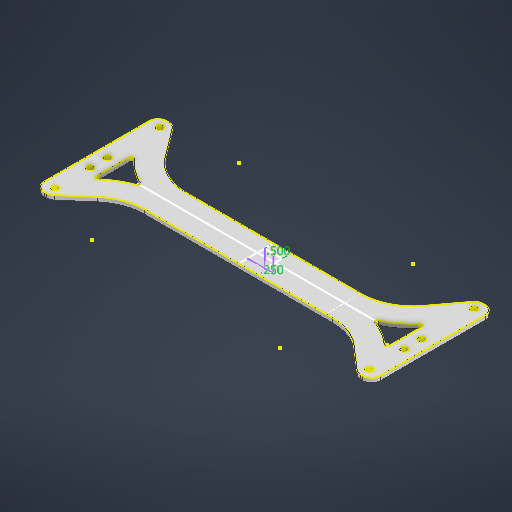
# Autodesk Inventor part: Lady Brown Arm Brace
Saved by Autodesk Inventor 2025 (Build 290162000, 162)
## iProperties
Created: 2024-12-31
Part Number: Lady Brown Arm Brace
Material: Generic
Document SubType Name: Modeling
Designer: Juan
Density: 1 g/cm^3
Appearance: Default
Author: Juan
Autodesk Inventor part; units mm, degrees
ref_plane "YZ Plane" through (0, 0, 0) normal (1, 0, 0) x (0, 1, 0)
ref_plane "XZ Plane" through (0, 0, 0) normal (0, 1, 0) x (-1, 0, 0)
ref_plane "XY Plane" through (0, 0, 0) normal (0, 0, 1) x (1, 0, 0)
sketch "Sketch1" plane through (0, 0, 0) normal (0, 1, 0) x (-1, 0, 0)
  line L0 (0, 0) -> (-114.3, 0)
  line L1 (0, 0) -> (114.3, 0)
  circle A0 centre (-114.3, 0) radius 2.3241
  circle A1 centre (114.3, 0) radius 2.3241
  line L2 (-114.3, 0) -> (-114.3, 12.7)
  line L3 (114.3, 0) -> (114.3, 12.7)
  circle A2 centre (114.3, 12.7) radius 2.3241
  circle A3 centre (-114.3, 12.7) radius 2.3241
  line L4 (114.3, 0) -> (122.2375, 0)
  line L5 (-114.3, 0) -> (-122.2375, 0)
  line L6 (-114.3, 12.7) -> (-122.2375, 12.7)
  line L7 (114.3, 12.7) -> (122.2375, 12.7)
  line L8 (-114.3, 0) -> (-114.3, -6.35)
  line L9 (-114.3, 12.7) -> (-114.3, 19.05)
  line L10 (114.3, 0) -> (114.3, -6.35)
  line L11 (114.3, 12.7) -> (114.3, 19.05)
  line L12 (122.2375, -6.35) -> (-122.2375, -6.35)
  line L13 (-122.2375, -6.35) -> (-122.2375, 19.05)
  line L14 (-122.2375, 19.05) -> (122.2375, 19.05)
  line L15 (122.2375, 19.05) -> (122.2375, -6.35)
  dimension "d0" = 114.3
  dimension "d1" = 114.3
  dimension "d2" = 4.6482
  dimension "d3" = 4.6482
  dimension "d4" = 12.7
  dimension "d5" = 12.7
  dimension "d6" = 4.6482
  dimension "d7" = 4.6482
  dimension "d8" = 7.9375
  dimension "d9" = 7.9375
  dimension "d10" = 6.35
  dimension "d11" = 6.35
  constraints: 32 end point, 7 horizontal, 6 vertical, 4 centre point, 4 coincident, 2 parallel, 1 perpendicular
  measures "d0" distance of L0.start L0.end
  measures "d1" distance of L0.start L1.end
  measures "d2" diameter of A0
  measures "d3" diameter of A1
  measures "d4" distance of L2.start L2.end
  measures "d5" distance of L3.start L3.end
  measures "d6" diameter of A2
  measures "d7" diameter of A3
  measures "d8" distance of L3.start L4.end
  measures "d9" distance of L2.start L5.end
  measures "d10" distance of L2.start L8.end
  measures "d11" distance of L6.start L9.end
extrude "Extrusion1" add sketch "Sketch1" along normal blind 3.175 contours L1 A1 L10 L12 L8 A0 L0 | L0 A0 L2 A3 L9 L14 L11 A2 L3 A1 L1 | A0 L5 L13 L6 A3 L2 | L8 L12 L13 L5 A0 | L3 A2 L7 L15 L4 A1 | A1 L4 L15 L12 L10 | L6 L13 L14 L9 A3 | L11 L14 L15 L7 A2
sketch "Sketch2" plane through (0, 3.175, 0) normal (0, 1, 0) x (1, 0, 0)
  circle A0 centre (114.3, -12.7) radius 2.3241 projected
  line L0 (0, 0) -> (0, -19.05)
  line L1 (-122.2375, -19.05) -> (122.2375, -19.05) projected
  line L2 (114.3, -12.7) -> (114.3, -38.1)
  circle A1 centre (114.3, -38.1) radius 2.3241
  line L3 (122.2375, -19.05) -> (107.95, -19.05)
  line L4 (107.95, -19.05) -> (107.95, -44.45)
  line L5 (107.95, -44.45) -> (122.2375, -44.45)
  line L6 (122.2375, -44.45) -> (122.2375, -19.05)
  circle A2 centre (114.3, 0) radius 2.3241 projected
  line L7 (114.3, 0) -> (114.3, 38.1)
  circle A3 centre (114.3, 38.1) radius 2.3241
  line L8 (122.2375, 6.35) -> (-122.2375, 6.35) projected
  line L9 (122.2375, 6.35) -> (107.95, 6.35)
  line L10 (107.95, 6.35) -> (107.95, 44.45)
  line L11 (107.95, 44.45) -> (122.2375, 44.45)
  line L12 (122.2375, 44.45) -> (122.2375, 6.35)
  line L13 (122.2375, -19.05) -> (122.2375, 6.35) projected
  circle A4 centre (-114.3, -38.1) radius 2.3241
  line L14 (-107.95, -19.05) -> (-107.95, -44.45)
  line L15 (-107.95, -44.45) -> (-122.2375, -44.45)
  line L16 (-122.2375, -44.45) -> (-122.2375, -19.05)
  circle A5 centre (-114.3, 38.1) radius 2.3241
  line L17 (-107.95, 6.35) -> (-107.95, 44.45)
  line L18 (-107.95, 44.45) -> (-122.2375, 44.45)
  line L19 (-122.2375, 44.45) -> (-122.2375, 6.35)
  line L20 (-122.2375, 6.35) -> (-122.2375, -19.05) projected
  dimension "d14" = 25.4
  dimension "d15" = 14.2875
  dimension "d16" = 25.4
  dimension "d17" = 38.1
  dimension "d18" = 4.6482
  dimension "d19" = 14.2875
  dimension "d20" = 38.1
  constraints: 34 end point, 8 symmetric about line, 4 centre point, 4 parallel, 2 coincident, 2 horizontal, 2 perpendicular, 2 vertical, 1 midpoint, 2 other
  measures "d14" distance of L2.start L2.end
  measures "d15" distance of L5.end L4.end
  measures "d16" distance of L5.end L1.end
  measures "d17" distance of L7.start L7.end
  measures "d18" diameter of A3
  measures "d19" distance of L10.end L11.end
  measures "d20" distance of L11.end L8.start
extrude "Extrusion2" add sketch "Sketch2" against normal blind 3.175 contours L1 L14 L15 L16 | L19 L18 L17 L8 | L1 L6 L5 L4 | L10 L11 L12 L8
fillet "Fillet1" radius 6.35 8 edges at (122.2375, 1.5875, 44.45) (107.95, 1.5875, 44.45) (122.2375, 1.5875, -44.45) (107.95, 1.5875, -44.45) (-107.95, 1.5875, 44.45) (-122.2375, 1.5875, 44.45) (-122.2375, 1.5875, -44.45) (-107.95, 1.5875, -44.45)
sketch "Sketch3" plane through (0, 3.175, 0) normal (0, 1, 0) x (1, 0, 0)
  line L0 (-107.95, -19.05) -> (107.95, -19.05) projected
  line L1 (107.95, -19.05) -> (107.95, -38.1) projected
  line L2 (-107.95, -38.1) -> (-107.95, -19.05) projected
  arc A0 (-114.3, -44.45) -> (-107.95, -38.1) centre (-114.3, -38.1) ccw projected
  arc A1 (107.95, -38.1) -> (114.3, -44.45) centre (114.3, -38.1) ccw projected
  line L3 (-107.95, -19.05) -> (107.95, -19.05) projected
  line L4 (107.95, -19.05) -> (82.55, -19.05)
  line L5 (82.55, -19.05) -> (110.1475, -42.9041)
  line L6 (0, 0) -> (0, -19.05)
  line L7 (107.95, 6.35) -> (-107.95, 6.35) projected
  line L8 (107.95, 6.35) -> (82.55, 6.35)
  arc A2 (114.3, 44.45) -> (107.95, 38.1) centre (114.3, 38.1) ccw projected
  line L9 (107.95, 38.1) -> (107.95, 6.35) projected
  line L10 (-107.95, 6.35) -> (-107.95, 38.1) projected
  arc A3 (-107.95, 38.1) -> (-114.3, 44.45) centre (-114.3, 38.1) ccw projected
  line L11 (82.55, 6.35) -> (109.22, 41.91)
  line L12 (-82.55, -19.05) -> (-110.1475, -42.9041)
  line L13 (-82.55, 6.35) -> (-109.22, 41.91)
  dimension "d24" = 25.4
  constraints: 14 end point, 4 symmetric about line, 2 point on circle, 2 point on line, 2 tangent, 1 midpoint
  measures "d24" distance of L0.end L4.end
extrude "Extrusion3" add sketch "Sketch3" against normal blind 3.175
fillet "Fillet2" radius 38.1 2 edges at (82.55, 1.5875, -6.35) (-82.55, 1.5875, -6.35)
fillet "Fillet3" radius 38.1 2 edges at (-82.55, 1.5875, 19.05) (82.55, 1.5875, 19.05)
sketch "Sketch4" plane through (0, 3.175, 0) normal (0, 1, 0) x (1, 0, 0)
  circle A0 centre (-114.3, 38.1) radius 2.3241 projected
  circle A1 centre (114.3, -38.1) radius 2.3241 projected
  circle A2 centre (-114.3, -38.1) radius 2.3241 projected
  circle A3 centre (114.3, 38.1) radius 2.3241 projected
  arc A4 (-109.22, 41.91) -> (-114.3, 44.45) centre (-114.3, 38.1) ccw projected
  line L0 (-114.3, 44.45) -> (-115.8875, 44.45) projected
  arc A5 (-115.8875, 44.45) -> (-122.2375, 38.1) centre (-115.8875, 38.1) ccw projected
  line L1 (-122.2375, 38.1) -> (-122.2375, -38.1) projected
  arc A6 (-122.2375, -38.1) -> (-115.8875, -44.45) centre (-115.8875, -38.1) ccw projected
  line L2 (-115.8875, -44.45) -> (-114.3, -44.45) projected
  arc A7 (-114.3, -44.45) -> (-110.1475, -42.9041) centre (-114.3, -38.1) ccw projected
  line L3 (-110.1475, -42.9041) -> (-93.2809, -28.3253) projected
  arc A8 (-68.3661, -19.05) -> (-93.2809, -28.3253) centre (-68.3661, -57.15) ccw projected
  line L4 (-68.3661, -19.05) -> (68.3661, -19.05) projected
  arc A9 (93.2809, -28.3253) -> (68.3661, -19.05) centre (68.3661, -57.15) ccw projected
  line L5 (93.2809, -28.3253) -> (110.1475, -42.9041) projected
  arc A10 (110.1475, -42.9041) -> (114.3, -44.45) centre (114.3, -38.1) ccw projected
  line L6 (114.3, -44.45) -> (115.8875, -44.45) projected
  arc A11 (115.8875, -44.45) -> (122.2375, -38.1) centre (115.8875, -38.1) ccw projected
  line L7 (122.2375, -38.1) -> (122.2375, 38.1) projected
  arc A12 (122.2375, 38.1) -> (115.8875, 44.45) centre (115.8875, 38.1) ccw projected
  line L8 (115.8875, 44.45) -> (114.3, 44.45) projected
  arc A13 (114.3, 44.45) -> (109.22, 41.91) centre (114.3, 38.1) ccw projected
  line L9 (109.22, 41.91) -> (93.98, 21.59) projected
  arc A14 (63.5, 6.35) -> (93.98, 21.59) centre (63.5, 44.45) ccw projected
  line L10 (63.5, 6.35) -> (-63.5, 6.35) projected
  arc A15 (-93.98, 21.59) -> (-63.5, 6.35) centre (-63.5, 44.45) ccw projected
  line L11 (-93.98, 21.59) -> (-109.22, 41.91) projected
  circle A16 centre (114.3, 0) radius 2.3241 projected
  circle A17 centre (-114.3, 0) radius 2.3241 projected
  circle A18 centre (-114.3, -12.7) radius 2.3241 projected
  circle A19 centre (114.3, -12.7) radius 2.3241 projected
  line L12 (-63.5, -9.174) -> (63.5, -9.174)
  arc A20 (63.5, -9.174) -> (106.3992, 12.2756) centre (63.5, 44.45) ccw
  line L13 (106.3992, 12.2756) -> (106.7135, 12.6946)
  line L14 (106.7135, 12.6946) -> (106.7135, -19.4165)
  line L15 (106.7135, -19.4165) -> (103.4325, -16.5806)
  arc A21 (103.4325, -16.5806) -> (68.3661, -3.526) centre (68.3661, -57.15) ccw
  line L16 (68.3661, -3.526) -> (-68.3661, -3.526)
  arc A22 (-68.3661, -3.526) -> (-103.4325, -16.5806) centre (-68.3661, -57.15) ccw
  line L17 (-103.4325, -16.5806) -> (-106.7135, -19.4165)
  line L18 (-106.7135, -19.4165) -> (-106.7135, 12.6946)
  line L19 (-106.7135, 12.6946) -> (-106.3992, 12.2756)
  arc A23 (-106.3992, 12.2756) -> (-63.5, -9.174) centre (-63.5, 44.45) ccw
  point P0 (0, 0)
  point P1 (82.9128, -5.5368)
  point P2 (-82.9128, -5.5368)
  constraints: 16 end point, 8 point on circle, 4 centre point, 11 other
extrude "Extrusion4" cut sketch "Sketch4" against normal blind 3.175 contours A22 L17 L18 L19 A23 | A20 L13 L14 L15 A21
fillet "Fillet4" radius 1.5875 6 edges at (-106.7135, 1.5875, -12.6946) (-106.7135, 1.5875, 19.4165) (-82.9128, 1.5875, 5.5368) (82.9128, 1.5875, 5.5368) (106.7135, 1.5875, 19.4165) (106.7135, 1.5875, -12.6946)
sketch "Sketch5" plane through (0, 3.175, 0) normal (0, 1, 0) x (1, 0, 0)
  arc A0 (106.7135, 8.179) -> (103.9291, 9.2219) centre (105.126, 8.179) ccw projected
  line L0 (106.7135, 8.179) -> (106.7135, -15.946) projected
  arc A1 (104.0879, -17.147) -> (106.7135, -15.946) centre (105.126, -15.946) ccw projected
  line L1 (104.0879, -17.147) -> (103.4325, -16.5806) projected
  arc A2 (103.4325, -16.5806) -> (86.8496, -6.8122) centre (68.3661, -57.15) ccw projected
  arc A3 (86.7097, -3.8909) -> (86.8496, -6.8122) centre (87.3968, -5.322) ccw projected
  arc A4 (86.7097, -3.8909) -> (103.9291, 9.2219) centre (63.5, 44.45) ccw projected
  line L2 (-103.4325, -16.5806) -> (-104.0879, -17.147) projected
  arc A5 (-106.7135, -15.946) -> (-104.0879, -17.147) centre (-105.126, -15.946) ccw projected
  line L3 (-106.7135, -15.946) -> (-106.7135, 8.179) projected
  arc A6 (-103.9291, 9.2219) -> (-106.7135, 8.179) centre (-105.126, 8.179) ccw projected
  arc A7 (-103.9291, 9.2219) -> (-86.7097, -3.8909) centre (-63.5, 44.45) ccw projected
  arc A8 (-86.8496, -6.8122) -> (-86.7097, -3.8909) centre (-87.3968, -5.322) ccw projected
  arc A9 (-86.8496, -6.8122) -> (-103.4325, -16.5806) centre (-68.3661, -57.15) ccw projected
  circle A10 centre (-114.3, 38.1) radius 2.3241 projected
  circle A11 centre (114.3, -38.1) radius 2.3241 projected
  circle A12 centre (-114.3, -38.1) radius 2.3241 projected
  circle A13 centre (114.3, 38.1) radius 2.3241 projected
  arc A14 (-109.22, 41.91) -> (-114.3, 44.45) centre (-114.3, 38.1) ccw projected
  line L4 (-114.3, 44.45) -> (-115.8875, 44.45) projected
  arc A15 (-115.8875, 44.45) -> (-122.2375, 38.1) centre (-115.8875, 38.1) ccw projected
  line L5 (-122.2375, 38.1) -> (-122.2375, -38.1) projected
  arc A16 (-122.2375, -38.1) -> (-115.8875, -44.45) centre (-115.8875, -38.1) ccw projected
  line L6 (-115.8875, -44.45) -> (-114.3, -44.45) projected
  arc A17 (-114.3, -44.45) -> (-110.1475, -42.9041) centre (-114.3, -38.1) ccw projected
  line L7 (-110.1475, -42.9041) -> (-93.2809, -28.3253) projected
  arc A18 (-68.3661, -19.05) -> (-93.2809, -28.3253) centre (-68.3661, -57.15) ccw projected
  line L8 (-68.3661, -19.05) -> (68.3661, -19.05) projected
  arc A19 (93.2809, -28.3253) -> (68.3661, -19.05) centre (68.3661, -57.15) ccw projected
  line L9 (93.2809, -28.3253) -> (110.1475, -42.9041) projected
  arc A20 (110.1475, -42.9041) -> (114.3, -44.45) centre (114.3, -38.1) ccw projected
  line L10 (114.3, -44.45) -> (115.8875, -44.45) projected
  arc A21 (115.8875, -44.45) -> (122.2375, -38.1) centre (115.8875, -38.1) ccw projected
  line L11 (122.2375, -38.1) -> (122.2375, 38.1) projected
  arc A22 (122.2375, 38.1) -> (115.8875, 44.45) centre (115.8875, 38.1) ccw projected
  line L12 (115.8875, 44.45) -> (114.3, 44.45) projected
  arc A23 (114.3, 44.45) -> (109.22, 41.91) centre (114.3, 38.1) ccw projected
  line L13 (109.22, 41.91) -> (93.98, 21.59) projected
  arc A24 (63.5, 6.35) -> (93.98, 21.59) centre (63.5, 44.45) ccw projected
  line L14 (63.5, 6.35) -> (-63.5, 6.35) projected
  arc A25 (-93.98, 21.59) -> (-63.5, 6.35) centre (-63.5, 44.45) ccw projected
  line L15 (-93.98, 21.59) -> (-109.22, 41.91) projected
  circle A26 centre (114.3, 0) radius 2.3241 projected
  circle A27 centre (-114.3, 0) radius 2.3241 projected
  circle A28 centre (-114.3, -12.7) radius 2.3241 projected
  circle A29 centre (114.3, -12.7) radius 2.3241 projected
  line L16 (-87.3968, -5.322) -> (87.3968, -5.322)
  line L17 (0, 0) -> (0, -12.7)
  line L18 (0, -19.05) -> (0, -12.7)
  line L19 (0, 6.35) -> (0, 0)
  line L20 (63.5, 6.35) -> (63.5, -19.05)
  line L21 (63.5, -19.05) -> (63.5, -12.7)
  line L22 (0, 0) -> (12.7, 0)
  line L23 (12.7, 0) -> (12.7, -12.7)
  line L24 (12.7, -12.7) -> (0, -12.7)
  line L25 (0, 0) -> (12.7, -12.7)
  line L26 (0, 0) -> (6.35, 0)
  line L27 (12.7, -12.7) -> (19.05, -12.7)
  line L28 (19.05, -12.7) -> (6.35, 0)
  dimension "d32" = 12.7
  dimension "d33" = 6.35
  constraints: 26 end point, 4 vertical, 3 horizontal, 3 midpoint, 2 perpendicular, 2 point on line
  measures "d32" distance of L17.start L22.end
  measures "d33" distance of L23.end L27.end
body "Solid1"
